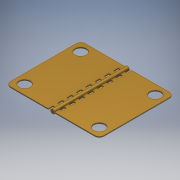
# Autodesk Inventor part: Scharnier
Saved by Autodesk Inventor 2018.3 (Build 223284000, 284)
## iProperties
Created: 2020-11-10
Part Number: Scharnier
Material: Generic
Document SubType Name: Modeling
Designer: daanv
Density: 1 g/cm^3
Appearance: Brass - Satin
Author: daanv
Autodesk Inventor part; units mm, degrees
ref_plane "YZ Plane" through (0, 0, 0) normal (1, 0, 0) x (0, 1, 0)
ref_plane "XZ Plane" through (0, 0, 0) normal (0, 1, 0) x (-1, 0, 0)
ref_plane "XY Plane" through (0, 0, 0) normal (0, 0, 1) x (1, 0, 0)
sketch "Sketch1" plane through (0, 0, 0) normal (0, 0, 1) x (1, 0, 0)
  line L0 (0, 0) -> (10, 0)
  line L1 (10, 0) -> (10, 8)
  line L2 (10, 8) -> (0, 8)
  line L3 (0, 8) -> (0, 0)
  dimension "d0" = 10
  dimension "d1" = 8
  constraints: 8 end point, 2 parallel, 1 horizontal, 1 perpendicular
  measures "d0" distance of L2.end L1.end
  measures "d1" distance of L1.end L0.end
extrude "Extrusion1" add sketch "Sketch1" along normal blind 0.1
sketch "Sketch2" plane through (0, 0, 0) normal (0, -1, 0) x (1, 0, 0)
  circle A0 centre (5, 0.05) radius 0.225
  dimension "d4" = 0.45
  constraints: 1 centre point
  measures "d4" diameter of A0
extrude "Extrusion2" add sketch "Sketch2" against normal blind 8
sketch "Sketch3" plane through (0, 0, 0.1) normal (0, 0, 1) x (1, 0, 0)
  point P0 (1, 7)
  point P1 (1, 1)
hole "Hole1" at (1, 7, 0.1) at (1, 1, 0.1) direction (0, 0, -1) diameter 1.2 end through all
sketch "Sketch4" plane through (0, 0, 0.1) normal (0, 0, 1) x (1, 0, 0)
  point P0 (0, 0)
  point P1 (9, 7)
  point P2 (9, 1)
hole "Hole2" at (9, 7, 0.1) at (9, 1, 0.1) direction (0, 0, -1) diameter 1.2 end through all
sketch "Sketch5" plane through (0, 0, 0.1) normal (0, 0, 1) x (1, 0, 0)
  line L0 (4.7806, 0) -> (4.7806, 8) projected
  line L1 (4.7806, 0) -> (4.5306, 0)
  line L2 (4.5306, 0) -> (4.5306, 0.5)
  line L3 (4.5306, 0.5) -> (4.7806, 0.5)
  line L4 (4.7806, 0.5) -> (4.7806, 0)
  line L5 (4.5306, 1) -> (4.7806, 1)
  line L6 (4.7806, 1) -> (4.7806, 1.5)
  line L7 (4.7806, 1.5) -> (4.5306, 1.5)
  line L8 (4.5306, 1.5) -> (4.5306, 1)
  line L9 (4.7806, 2) -> (4.5306, 2)
  line L10 (4.5306, 2) -> (4.5306, 2.5)
  line L11 (4.5306, 2.5) -> (4.7806, 2.5)
  line L12 (4.7806, 2.5) -> (4.7806, 2)
  line L13 (4.7806, 3) -> (4.5306, 3)
  line L14 (4.5306, 3) -> (4.5306, 3.5)
  line L15 (4.5306, 3.5) -> (4.7806, 3.5)
  line L16 (4.7806, 3.5) -> (4.7806, 3)
  line L17 (4.7806, 4) -> (4.5306, 4)
  line L18 (4.5306, 4) -> (4.5306, 4.5)
  line L19 (4.5306, 4.5) -> (4.7806, 4.5)
  line L20 (4.7806, 4.5) -> (4.7806, 4)
  line L21 (4.7806, 5) -> (4.5306, 5)
  line L22 (4.5306, 5) -> (4.5306, 5.5)
  line L23 (4.5306, 5.5) -> (4.7806, 5.5)
  line L24 (4.7806, 5.5) -> (4.7806, 5)
  line L25 (4.7806, 6) -> (4.5306, 6)
  line L26 (4.5306, 6) -> (4.5306, 6.5)
  line L27 (4.5306, 6.5) -> (4.7806, 6.5)
  line L28 (4.7806, 6.5) -> (4.7806, 6)
  line L29 (4.7806, 7) -> (4.5306, 7)
  line L30 (4.5306, 7) -> (4.5306, 7.5)
  line L31 (4.5306, 7.5) -> (4.7806, 7.5)
  line L32 (4.7806, 7.5) -> (4.7806, 7)
  dimension "d21" = 0.25
  dimension "d22" = 0.5
  dimension "d23" = 0.5
  dimension "d24" = 0.5
  dimension "d25" = 0.5
  dimension "d26" = 0.5
  dimension "d27" = 0.5
  dimension "d28" = 0.5
  dimension "d29" = 0.5
  constraints: 64 end point, 16 parallel, 8 horizontal, 8 perpendicular, 6 point on line, 8 other
  measures "d21" distance of L2.end L3.end
  measures "d22" distance of L1.end L2.end
  measures "d23" distance of L6.end L5.end
  measures "d24" distance of L9.end L10.end
  measures "d25" distance of L13.end L14.end
  measures "d26" distance of L17.end L18.end
  measures "d27" distance of L21.end L22.end
  measures "d28" distance of L25.end L26.end
  measures "d29" distance of L29.end L30.end
extrude "Extrusion3" cut sketch "Sketch5" against normal blind 8
sketch "Sketch6" plane through (0, 0, 0.1) normal (0, 0, 1) x (1, 0, 0)
  line L0 (10, 8) -> (5.2194, 8) projected
  line L1 (5.2194, 0) -> (5.2194, 8) projected
  line L2 (5.2194, 0.5) -> (5.4694, 0.5)
  line L3 (5.4694, 0.5) -> (5.4694, 1)
  line L4 (5.4694, 1) -> (5.2194, 1)
  line L5 (5.2194, 1) -> (5.2194, 0.5)
  line L6 (5.2194, 1.5) -> (5.4694, 1.5)
  line L7 (5.4694, 1.5) -> (5.4694, 2)
  line L8 (5.4694, 2) -> (5.2194, 2)
  line L9 (5.2194, 2) -> (5.2194, 1.5)
  line L10 (5.2194, 2.5) -> (5.4694, 2.5)
  line L11 (5.4694, 2.5) -> (5.4694, 3)
  line L12 (5.4694, 3) -> (5.2194, 3)
  line L13 (5.2194, 3) -> (5.2194, 2.5)
  line L14 (5.2194, 3.5) -> (5.4694, 3.5)
  line L15 (5.4694, 3.5) -> (5.4694, 4)
  line L16 (5.4694, 4) -> (5.2194, 4)
  line L17 (5.2194, 4) -> (5.2194, 3.5)
  line L18 (5.2194, 4.5) -> (5.4694, 4.5)
  line L19 (5.4694, 4.5) -> (5.4694, 5)
  line L20 (5.4694, 5) -> (5.2194, 5)
  line L21 (5.2194, 5) -> (5.2194, 4.5)
  line L22 (5.2194, 5.5) -> (5.4694, 5.5)
  line L23 (5.4694, 5.5) -> (5.4694, 6)
  line L24 (5.4694, 6) -> (5.2194, 6)
  line L25 (5.2194, 6) -> (5.2194, 5.5)
  line L26 (5.2194, 6.5) -> (5.4694, 6.5)
  line L27 (5.4694, 6.5) -> (5.4694, 7)
  line L28 (5.4694, 7) -> (5.2194, 7)
  line L29 (5.2194, 7) -> (5.2194, 6.5)
  line L30 (5.2194, 7.5) -> (5.4694, 7.5)
  line L31 (5.4694, 7.5) -> (5.4694, 8)
  line L32 (5.4694, 8) -> (5.2194, 8)
  line L33 (5.2194, 8) -> (5.2194, 7.5)
  point P0 (0, 0)
  dimension "d32" = 0.25
  dimension "d33" = 0.5
  dimension "d36" = 0.5
  dimension "d37" = 0.5
  dimension "d38" = 0.5
  dimension "d39" = 0.5
  dimension "d40" = 0.5
  dimension "d41" = 0.5
  constraints: 64 end point, 16 parallel, 8 horizontal, 8 perpendicular, 7 point on line, 9 other
  measures "d32" distance of L4.end L3.end
  measures "d33" distance of L3.end L2.end
  measures "d36" distance of L7.end L6.end
  measures "d37" distance of L11.end L10.end
  measures "d38" distance of L15.end L14.end
  measures "d39" distance of L19.end L18.end
  measures "d40" distance of L23.end L22.end
  measures "d41" distance of L27.end L26.end
extrude "Extrusion4" cut sketch "Sketch6" against normal blind 8
fillet "Fillet1" radius 0.5 4 edges at (0, 0, 0.05) (0, 8, 0.05) (10, 8, 0.05) (10, 0, 0.05)
body "Solid1"
